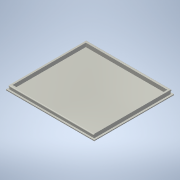
# Autodesk Inventor part: BARB_bottom
Saved by Autodesk Inventor 2022.3 (Build 263350000, 350)
## iProperties
Created: 2022-06-21
Part Number: BARB_bottom
Material: ABS Plastic
Document SubType Name: Modeling
Designer: abmos
Density: 1.06 g/cm^3
Appearance: Smooth - Ivory
Author: abmos
Autodesk Inventor part; units mm, degrees
ref_plane "YZ Plane" through (0, 0, 0) normal (1, 0, 0) x (0, 1, 0)
ref_plane "XZ Plane" through (0, 0, 0) normal (0, 1, 0) x (-1, 0, 0)
ref_plane "XY Plane" through (0, 0, 0) normal (0, 0, 1) x (1, 0, 0)
sketch "Master_XZ" plane through (0, 0, 0) normal (0, 1, 0) x (-1, 0, 0)
  line L0 (52.5, 47.5) -> (-52.5, 47.5)
  line L1 (-52.5, 47.5) -> (-52.5, -47.5)
  line L2 (-52.5, -47.5) -> (52.5, -47.5)
  line L3 (52.5, -47.5) -> (52.5, 47.5)
  line L4 (52.5, 47.5) -> (-52.5, -47.5) construction
  line L5 (-52.5, 47.5) -> (52.5, -47.5) construction
  line L6 (50.5, 45.5) -> (-50.5, 45.5)
  line L7 (-50.5, 45.5) -> (-50.5, -45.5)
  line L8 (-50.5, -45.5) -> (50.5, -45.5)
  line L9 (50.5, -45.5) -> (50.5, 45.5)
  line L10 (48.5, 43.5) -> (-48.5, 43.5)
  line L11 (-48.5, 43.5) -> (-48.5, -43.5)
  line L12 (-48.5, -43.5) -> (48.5, -43.5)
  line L13 (48.5, -43.5) -> (48.5, 43.5)
  point P0 (0, 0)
  dimension "d0" = 2
  dimension "d1" = 2
  dimension "d10" = 105
  dimension "d15" = 95
  constraints: 28 end point, 6 parallel, 3 perpendicular, 2 midpoint, 1 horizontal, 6 other
  measures "d0" distance between parallel lines of L3 L9
  measures "d1" distance between parallel lines of L9 L13
  measures "d10" distance of L0.start L0.end
  measures "d15" distance of L2.end L0.start
extrude "Floor" add sketch "Master_XZ" along normal blind 2 contours L3 L2 L1 L0 | L9 L8 L7 L6 | L13 L12 L11 L10
extrude "Walls" add sketch "Master_XZ" along normal blind 6 contours L9 L8 L7 L6
sketch "Lip_profile" plane through (0, 1, -41.5) normal (1, 0, 0) x (0, 0, -1)
  line L0 (-87, 1) -> (-87, 5) projected
  circle A0 centre (-87, 4) radius 1
  line L1 (-87, 5) -> (4, 5) projected
  line L2 (-87, 5) -> (-87, 3)
  point P0 (-41.5, -1)
  dimension "d6" = 2
  dimension "d7" = 1
  constraints: 2 end point, 1 midpoint, 1 point on line, 3 other
  measures "d7" distance from line of L1 point (-87, 4)
extrude "Lip" add sketch "Lip_profile" along normal mid plane 100
sketch "Sketch3" plane through (50, 1, -41.5) normal (1, 0, 0) x (0, 0, -1)
  line L0 (-87, 5) -> (-87, 3) projected
  line L1 (-87, 5) -> (-87, 3) projected
  arc A0 (-87, 5) -> (-87, 3) centre (-87, 4) ccw projected
  point P0 (-41.5, -1)
revolve "Lip_edge_right" add sketch "Sketch3" angle 90 about axis through (50, 6, 45.5) along (0, 1, 0)
sketch "Sketch4" plane through (-50, 1, -41.5) normal (-1, 0, 0) x (0, 0, 1)
  line L0 (87, 3) -> (87, 5) projected
  arc A0 (87, 3) -> (87, 5) centre (87, 4) ccw projected
  point P0 (41.5, -1)
revolve "Lip_edge_left" add sketch "Sketch4" angle 90 about axis through (-50, 4, 45.5) along (0, -1, 0)
pattern_circular "Circular Pattern1" count 2 over 360 about axis through (0, -10, 0) along (0, 1, 0) of "Lip", "Lip_edge_right", "Lip_edge_left"
